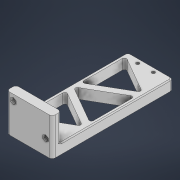
# Autodesk Inventor part: valve_fittter
Saved by Autodesk Inventor 2022 (Build 260153000, 153)
## iProperties
Created: 2023-06-08
Part Number: valve_fittter
Material: Generic
Document SubType Name: Modeling
Designer: Jakob Saugbjerg
Density: 1 g/cm^3
Appearance: Default
Author: Jakob Saugbjerg
Autodesk Inventor part; units mm, degrees
ref_plane "YZ Plane" through (0, 0, 0) normal (1, 0, 0) x (0, 1, 0)
ref_plane "XZ Plane" through (0, 0, 0) normal (0, 1, 0) x (-1, 0, 0)
ref_plane "XY Plane" through (0, 0, 0) normal (0, 0, 1) x (1, 0, 0)
sketch "Sketch1" plane through (0, 0, 0) normal (0, 0, 1) x (1, 0, 0)
  line L0 (0, 0) -> (45, 0)
  line L1 (45, 0) -> (45, 10)
  line L2 (45, 10) -> (0, 10)
  line L3 (0, 10) -> (0, 0)
  dimension "d0" = 45
  dimension "d1" = 10
  constraints: 8 end point, 2 parallel, 1 horizontal, 1 perpendicular
  measures "d0" distance of L2.end L1.end
  measures "d1" distance of L1.end L0.end
extrude "Extrusion1" add sketch "Sketch1" along normal blind 120
sketch "Sketch2" plane through (0, 10, 0) normal (0, 1, 0) x (1, 0, 0)
  line L0 (45, -120) -> (0, -120) projected
  line L1 (45, 0) -> (45, -120) projected
  line L2 (0, -120) -> (45, -120)
  line L3 (45, -120) -> (45, -111)
  line L4 (45, -111) -> (0, -111)
  line L5 (0, -111) -> (0, -120)
  point P0 (0, 0)
  dimension "d4" = 9
  constraints: 8 end point, 2 parallel, 1 horizontal, 1 perpendicular, 1 point on line
  measures "d4" distance of L3.end L2.end
extrude "Extrusion2" add sketch "Sketch2" along normal blind 27
sketch "Sketch3" plane through (45, 10, 111) normal (0, 0, -1) x (-1, 0, 0)
  line L0 (0, 0) -> (45, 0) projected
  line L1 (0, 0) -> (6.5, 0)
  line L2 (6.5, 0) -> (6.5, 5)
  line L3 (6.5, 5) -> (0, 5)
  line L4 (0, 5) -> (0, 0)
  circle A0 centre (6.5, 5) radius 1.6
  line L5 (6.5, 5) -> (6.5, 21)
  line L6 (6.5, 21) -> (38.5, 21)
  circle A1 centre (38.5, 21) radius 1.6
  point P0 (45, -10)
  dimension "d7" = 6.5
  dimension "d8" = 5
  dimension "d9" = 3.2
  dimension "d10" = 16
  dimension "d11" = 32
  dimension "d12" = 3.2
  constraints: 12 end point, 2 centre point, 2 coincident, 2 parallel, 2 perpendicular, 1 horizontal, 1 vertical
  measures "d7" distance of L3.end L2.end
  measures "d8" distance of L2.end L1.end
  measures "d9" diameter of A0
  measures "d10" distance of L5.start L5.end
  measures "d11" distance of L5.end L6.end
  measures "d12" diameter of A1
extrude "Extrusion3" cut sketch "Sketch3" against normal blind 27 contours A0 L3 L2 | L2 L5 A0 | A0 L5 L3 | A1
sketch "Sketch4" plane through (0, 0, 120) normal (0, 0, 1) x (1, 0, 0)
  circle A0 centre (6.5, 31) radius 1.6 projected
  line L0 (6.5, 31) -> (9.25, 31)
  circle A1 centre (38.5, 15) radius 1.6 projected
  line L1 (38.5, 15) -> (35.75, 15)
  line L2 (9.25, 29.4123) -> (6.5, 27.8246)
  line L3 (6.5, 27.8246) -> (3.75, 29.4123)
  line L4 (3.75, 29.4123) -> (3.75, 32.5877)
  line L5 (3.75, 32.5877) -> (6.5, 34.1754)
  line L6 (6.5, 34.1754) -> (9.25, 32.5877)
  line L7 (9.25, 32.5877) -> (9.25, 29.4123)
  line L8 (35.75, 16.5877) -> (38.5, 18.1754)
  line L9 (38.5, 18.1754) -> (41.25, 16.5877)
  line L10 (41.25, 16.5877) -> (41.25, 13.4123)
  line L11 (41.25, 13.4123) -> (38.5, 11.8246)
  line L12 (38.5, 11.8246) -> (35.75, 13.4123)
  line L13 (35.75, 13.4123) -> (35.75, 16.5877)
  point P0 (0, 0)
  dimension "d15" = 2.75
  dimension "d16" = 2.75
  constraints: 28 end point, 2 coincident, 2 horizontal, 2 midpoint, 26 other
  measures "d15" distance of L0.start L0.end
  measures "d16" distance of L1.start L1.end
extrude "Extrusion4" cut sketch "Sketch4" against normal blind 2.7 contours A0 | A1 | L2 L3 L4 L5 L6 L7 | L8 L9 L10 L11 L12 L13
sketch "Sketch5" plane through (0, 10, 0) normal (0, 1, 0) x (1, 0, 0)
  line L0 (45, 0) -> (0, 0) projected
  line L1 (22.5, 0) -> (22.5, -5)
  line L2 (22.5, -5) -> (14.75, -5)
  line L3 (14.75, -5) -> (30.25, -5)
  circle A0 centre (14.75, -5) radius 1.6
  circle A1 centre (30.25, -5) radius 1.6
  dimension "d19" = 5
  dimension "d20" = 7.75
  dimension "d21" = 15.5
  dimension "d22" = 3.2
  dimension "d23" = 3.2
  constraints: 6 end point, 2 centre point, 2 coincident, 1 midpoint, 1 perpendicular, 1 point on line, 1 vertical
  measures "d19" distance of L1.start L1.end
  measures "d20" distance of L1.end L2.end
  measures "d21" distance of L2.end L3.end
  measures "d22" diameter of A0
  measures "d23" diameter of A1
extrude "Extrusion5" cut sketch "Sketch5" against normal blind 10
sketch "Sketch7" plane through (0, 0, 0) normal (0, -1, 0) x (1, 0, 0)
  circle A0 centre (14.75, 5) radius 1.6 projected
  circle A1 centre (14.75, 5) radius 2.95
  circle A2 centre (30.25, 5) radius 1.6 projected
  circle A3 centre (30.25, 5) radius 2.95
  point P0 (0, 0)
  dimension "d30" = 5.9
  dimension "d31" = 5.9
  constraints: 2 centre point, 2 coincident
  measures "d30" diameter of A1
  measures "d31" diameter of A3
extrude "Extrusion7" cut sketch "Sketch7" against normal blind 5
fillet "Fillet1" radius 3 2 edges at (45, 5, 0) (0, 5, 0)
fillet "Fillet2" radius 3 4 edges at (45, 18.5, 120) (0, 18.5, 120) (45, 23.5, 111) (0, 23.5, 111)
chamfer "Chamfer1" distance 0.5 angle 45 3 edges at (22.5, 10, 111) (44.1213, 10, 111.8787) (0.8787, 10, 111.8787)
chamfer "Chamfer2" distance 1 angle 45 7 edges at (45, 10, 111.5986) (45, 10, 57) (44.1213, 10, 0.8787) (22.5, 10, 0) (0.8787, 10, 0.8787) (0, 10, 111.5986) (0, 10, 57)
sketch "Sketch8" plane through (3, 10, 110.5) normal (0, 1, 0) x (1, 0, 0)
  line L0 (39, 110.5) -> (0, 110.5) projected
  line L1 (0, 110.5) -> (0, 105.5)
  line L2 (0, 105.5) -> (28.496, 105.5) construction
  line L3 (42, -0.1459) -> (42, 107.5) projected
  line L4 (42, 78.3399) -> (39, 78.3399)
  line L5 (42, 78.3399) -> (45, 78.3399) construction
  line L6 (39, 78.3399) -> (39, 102.6874)
  line L7 (39, 102.6874) -> (39, 59.0142)
  line L8 (3, 103.7679) -> (36, 84.7154)
  line L9 (0, 105.5) -> (38.1051, 105.5) construction
  line L10 (36, 81.2513) -> (3, 62.1987)
  line L11 (0, 63.9308) -> (0, 102.0359)
  line L12 (39, 82.9833) -> (39, 75.9833)
  line L13 (36, 74.2513) -> (3, 55.1987)
  line L14 (3, 51.7346) -> (36, 32.6821)
  line L15 (39, 34.4141) -> (39, 72.5192)
  arc A0 (3, 55.1987) -> (3, 51.7346) centre (4, 53.4667) ccw
  arc A1 (36, 32.6821) -> (39, 34.4141) centre (37, 34.4141) ccw
  arc A2 (39, 72.5192) -> (36, 74.2513) centre (37, 72.5192) ccw
  arc A3 (0, 63.9308) -> (3, 62.1987) centre (2, 63.9308) ccw
  arc A4 (3, 103.7679) -> (0, 102.0359) centre (2, 102.0359) ccw
  arc A5 (36, 81.2513) -> (36, 84.7154) centre (35, 82.9833) ccw
  line L16 (0, 53.4667) -> (0, 46.4667)
  line L17 (-2, -0.6277) -> (-2, 107.5) projected
  line L18 (0, 53.4667) -> (7, 53.4667) construction
  line L19 (0, 46.4667) -> (38.1051, 46.4667) construction
  line L20 (-3, 107.5) -> (-3, -0.1459) projected
  line L21 (0, 46.4667) -> (38.4226, 24.2834)
  line L22 (0, 46.4667) -> (44.3667, 46.4667) construction
  line L23 (38.4226, 24.2834) -> (0, 2.1)
  line L24 (0, 2.1) -> (0, 46.4667)
  point P0 (-3, 110.5)
  dimension "d42" = 5
  dimension "d44" = 3
  dimension "d45" = 180
  dimension "d47" = 30
  dimension "d48" = 60
  dimension "d49" = 7
  dimension "d50" = 120
  dimension "d51" = 60
  dimension "d52" = 2
  dimension "d55" = 7
  dimension "d56" = 90
  dimension "d64" = 30
  dimension "d65" = 60
  constraints: 42 end point, 13 point on line, 12 point on circle, 12 tangent, 6 centre point, 6 horizontal, 5 equal radius, 4 equal length, 3 parallel, 2 vertical, 1 collinear, 1 perpendicular
  measures "d42" distance of L0.end L1.end
  measures "d44" distance of L4.start L4.end
  measures "d45" angle of L4 L5
  measures "d47" angle of L8 L9
  measures "d48" angle of L8 L10
  measures "d49" distance of L12.start L12.end
  measures "d50" angle of L12 L13
  measures "d51" angle of L14 L13
  measures "d52" radius of A0
  measures "d55" distance of L16.start L16.end
  measures "d56" angle of L16 L18
  measures "d64" angle of L21 L22
  measures "d65" angle of L21 L23
extrude "Extrusion8" cut sketch "Sketch8" against normal blind 10
fillet "Fillet3" radius 2 3 edges at (41.4226, 5, 86.2166) (3, 5, 64.0333) (3, 5, 108.4)
body "Solid1"
